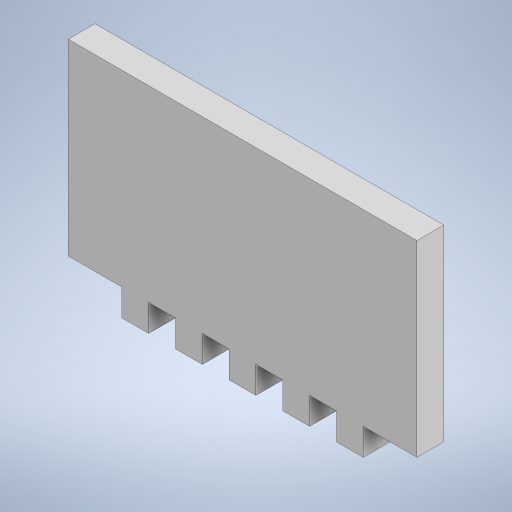
# Autodesk Inventor part: backside
Saved by Autodesk Inventor 2024 (Build 280153000, 153)
## iProperties
Created: 2024-04-15
Part Number: backside
Material: Generic
Document SubType Name: Modeling
Designer: srika
Density: 1 g/cm^3
Appearance: Default
Author: srika
Autodesk Inventor part; units mm, degrees
ref_plane "YZ Plane" through (0, 0, 0) normal (1, 0, 0) x (0, 1, 0)
ref_plane "XZ Plane" through (0, 0, 0) normal (0, 1, 0) x (-1, 0, 0)
ref_plane "XY Plane" through (0, 0, 0) normal (0, 0, 1) x (1, 0, 0)
sketch "Sketch2" plane through (0, 0, 0) normal (0, 0, 1) x (1, 0, 0)
  line L0 (5, 5) -> (70, 5)
  line L1 (70, 5) -> (70, 40)
  line L2 (70, 40) -> (5, 40)
  line L3 (5, 40) -> (5, 5)
  line L4 (15, 5) -> (20, 5)
  line L5 (20, 5) -> (20, 0)
  line L6 (20, 0) -> (15, 0)
  line L7 (15, 0) -> (15, 5)
  line L8 (30, 5) -> (30, 0)
  line L9 (30, 0) -> (25, 0)
  line L10 (25, 0) -> (25, 5)
  line L11 (40, 5) -> (40, 0)
  line L12 (40, 0) -> (35, 0)
  line L13 (35, 0) -> (35, 5)
  line L14 (50, 5) -> (50, 0)
  line L15 (50, 0) -> (45, 0)
  line L16 (45, 0) -> (45, 5)
  line L17 (60, 5) -> (60, 0)
  line L18 (60, 0) -> (55, 0)
  line L19 (55, 0) -> (55, 5)
  line L20 (70, 35) -> (75, 35)
  line L21 (75, 35) -> (75, 30)
  line L22 (75, 30) -> (70, 30)
  line L23 (70, 30) -> (70, 35)
  line L24 (75, 20) -> (70, 20)
  line L25 (70, 25) -> (75, 25)
  line L26 (75, 25) -> (75, 20)
  line L27 (75, 10) -> (70, 10)
  line L28 (70, 15) -> (75, 15)
  line L29 (75, 15) -> (75, 10)
  dimension "d122" = 10
  dimension "d129" = 65
  dimension "d132" = 10
  constraints: 60 end point, 6 parallel, 4 horizontal, 3 perpendicular, 1 point on line, 1 vertical, 42 other
  measures "d122" distance of L5.end L8.end
  measures "d129" distance of L1.end L2.end
  measures "d132" distance of L21.end L24.start
extrude "Extrusion4" add sketch "Sketch2" along normal blind 5 contours L3 L2 L1 L0 | L0 L5 L6 L7 | L0 L8 L9 L10 | L0 L11 L12 L13 | L0 L14 L15 L16 | L0 L17 L18 L19
body "Solid4"
